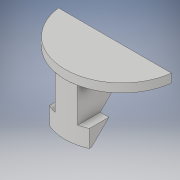
# Autodesk Inventor part: BUTTON_INSIDE
Saved by Autodesk Inventor 2019 (Build 230136000, 136)
## iProperties
Created: 2018-12-19
Part Number: BUTTON_INSIDE
Material: Типовые
Document SubType Name: Modeling
Designer: aldanstar
Density: 1 g/cm^3
Appearance: По умолчанию
Author: aldanstar
Autodesk Inventor part; units mm, degrees
ref_plane "YZ Plane" through (0, 0, 0) normal (1, 0, 0) x (0, 1, 0)
ref_plane "XZ Plane" through (0, 0, 0) normal (0, 1, 0) x (-1, 0, 0)
ref_plane "XY Plane" through (0, 0, 0) normal (0, 0, 1) x (1, 0, 0)
sketch "Эскиз1" plane through (0, 0, 0) normal (0, 1, 0) x (-1, 0, 0)
  line L0 (2.3, 2.625) -> (-2.3, 2.625) construction
  line L1 (-2.3, 2.625) -> (-2.3, -2.625)
  line L2 (-2.3, -2.625) -> (2.3, -2.625)
  line L3 (2.3, -2.625) -> (2.3, 2.625)
  line L4 (3.22, 0) -> (-3.22, 0) projected
  line L5 (0, -3.7758) -> (0, 4.2798) projected
  arc A0 (2.3, 2.625) -> (-2.3, 2.625) centre (0, -2.371) ccw
  point P0 (0, 0)
  dimension "d0" = 4.6
  dimension "d10" = 5.25
  dimension "d17" = 5.5
  constraints: 8 end point, 2 parallel, 2 point on circle, 1 centre point, 1 horizontal, 1 perpendicular, 2 other
  measures "d0" distance of L1.end L2.end
  measures "d10" distance of L2.end L0.start
  measures "d17" radius of A0
extrude "Выдавливание1" add sketch "Эскиз1" along normal blind 5
chamfer "Фаска2" distance 5 angle 45 1 edges at (0, 0, -2.625)
sketch "Эскиз3" plane through (0, 5, 0) normal (0, 1, 0) x (1, 0, 0)
  line L0 (2.3, -2.625) -> (2.3, 2.625) projected
  line L1 (2.3, 2.625) -> (1.3, 2.625)
  line L2 (1.3, 2.625) -> (1.3, -3.129)
  line L3 (1.3, -3.129) -> (2.3, -3.129)
  line L4 (2.3, -3.129) -> (2.3, 2.625)
  arc A0 (-2.3, -2.625) -> (2.3, -2.625) centre (0, 2.371) ccw projected
  point P0 (0, 0)
  dimension "d14" = 1
  constraints: 8 end point, 2 horizontal, 2 parallel, 1 perpendicular, 1 other
  measures "d14" distance between parallel lines of L0 L2
extrude "Выдавливание3" cut sketch "Эскиз3" against normal blind 3
mirror "Зеркальное отражение1" about plane through (0, 0, 0) normal (1, 0, 0) of "Выдавливание3"
sketch "Эскиз4" plane through (0, 5, 0) normal (0, 1, 0) x (1, 0, 0)
  line L0 (-1.3, 2.625) -> (-1.3, -2.9732) projected
  arc A0 (-1.3, -2.9732) -> (1.3, -2.9732) centre (0, 2.371) ccw projected
  line L1 (1.3, -2.9732) -> (1.3, 2.625) projected
  line L2 (1.3, 2.625) -> (-1.3, 2.625) projected
  point P0 (0, 0)
extrude "Выдавливание4" add sketch "Эскиз4" along normal blind 1
sketch "Эскиз5" plane through (0, 6, 0) normal (0, 1, 0) x (1, 0, 0)
  line L0 (6.5, 2.625) -> (-6.5, 2.625)
  line L1 (1.3, 2.625) -> (-1.3, 2.625) projected
  line L2 (0, 4.729) -> (0, -4.4387) projected
  arc A0 (-6.5, 2.625) -> (6.5, 2.625) centre (0, 3.4194) ccw
  arc A1 (-1.3, -2.9732) -> (1.3, -2.9732) centre (0, 2.371) ccw projected
  point P0 (0, 0)
  point P1 (0, -3.129)
  dimension "d20" = 13
  constraints: 4 point on circle, 2 end point, 1 centre point, 1 collinear, 1 horizontal, 1 symmetric about line
  measures "d20" distance of L0.start L0.end
extrude "Выдавливание5" add sketch "Эскиз5" along normal blind 1
